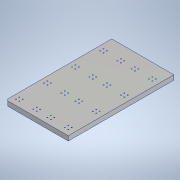
# Autodesk Inventor part: Assembly Plate
Saved by Autodesk Inventor 2022 (Build 260153000, 153)
## iProperties
Created: 2021-01-11
Part Number: Assembly Plate
Material: Aluminum 6061
Document SubType Name: Modeling
Designer: caleb
Density: 2.7 g/cm^3
Appearance: Aluminum - Flat
Author: caleb
Autodesk Inventor part; units mm, degrees
ref_plane "YZ Plane" through (0, 0, 0) normal (1, 0, 0) x (0, 1, 0)
ref_plane "XZ Plane" through (0, 0, 0) normal (0, 1, 0) x (-1, 0, 0)
ref_plane "XY Plane" through (0, 0, 0) normal (0, 0, 1) x (1, 0, 0)
sketch "Sketch1" plane through (0, 0, 0) normal (0, 1, 0) x (-1, 0, 0)
  line L0 (-63.5, 107.95) -> (63.5, 107.95)
  line L1 (63.5, 107.95) -> (63.5, -107.95)
  line L2 (63.5, -107.95) -> (-63.5, -107.95)
  line L3 (-63.5, -107.95) -> (-63.5, 107.95)
  line L4 (-63.5, 107.95) -> (63.5, -107.95) construction
  line L5 (63.5, 107.95) -> (-63.5, -107.95) construction
  point P0 (0, 0)
  dimension "d0" = 127
  dimension "d1" = 215.9
  constraints: 12 end point, 2 midpoint, 2 parallel, 1 horizontal, 1 perpendicular
  measures "d0" distance of L1.end L2.end
  measures "d1" distance of L0.end L1.end
extrude "Extrusion1" add sketch "Sketch1" along normal blind 9.525
chamfer "Chamfer1" distance 3.175 angle 45 1 edges at (-63.5, 4.7625, 107.95)
sketch "Sketch10" plane through (0, 9.525, 0) normal (0, 1, 0) x (1, 0, 0)
  circle A0 centre (-54.5, -96.95) radius 1
  circle A1 centre (-54.5, -89.95) radius 1
  circle A2 centre (-47.5, -96.95) radius 1
  circle A3 centre (-47.5, -89.95) radius 1
  line L0 (-63.5, 107.95) -> (-63.5, -104.775) projected
  line L1 (-60.325, -107.95) -> (63.5, -107.95) projected
  circle A4 centre (-54.5, -39.633) radius 1
  circle A5 centre (-54.5, -32.633) radius 1
  circle A6 centre (-47.5, -39.633) radius 1
  circle A7 centre (-47.5, -32.633) radius 1
  circle A8 centre (-54.5, 17.684) radius 1
  circle A9 centre (-54.5, 24.684) radius 1
  circle A10 centre (-47.5, 17.684) radius 1
  circle A11 centre (-47.5, 24.684) radius 1
  circle A12 centre (-54.5, 75.001) radius 1
  circle A13 centre (-54.5, 82.001) radius 1
  circle A14 centre (-47.5, 75.001) radius 1
  circle A15 centre (-47.5, 82.001) radius 1
  circle A16 centre (-18.934, -96.95) radius 1
  circle A17 centre (-18.934, -89.95) radius 1
  circle A18 centre (-11.934, -96.95) radius 1
  circle A19 centre (-11.934, -89.95) radius 1
  circle A20 centre (-18.934, -39.633) radius 1
  circle A21 centre (-18.934, -32.633) radius 1
  circle A22 centre (-11.934, -39.633) radius 1
  circle A23 centre (-11.934, -32.633) radius 1
  circle A24 centre (-18.934, 17.684) radius 1
  circle A25 centre (-18.934, 24.684) radius 1
  circle A26 centre (-11.934, 17.684) radius 1
  circle A27 centre (-11.934, 24.684) radius 1
  circle A28 centre (-18.934, 75.001) radius 1
  circle A29 centre (-18.934, 82.001) radius 1
  circle A30 centre (-11.934, 75.001) radius 1
  circle A31 centre (-11.934, 82.001) radius 1
  circle A32 centre (52.5, -96.95) radius 1
  circle A33 centre (45.5, -96.95) radius 1
  circle A34 centre (45.5, -89.95) radius 1
  circle A35 centre (52.5, -89.95) radius 1
  line L2 (63.5, -107.95) -> (63.5, 107.95) projected
  circle A36 centre (45.5, -32.633) radius 1
  circle A37 centre (45.5, -39.633) radius 1
  circle A38 centre (52.5, -39.633) radius 1
  circle A39 centre (52.5, -32.633) radius 1
  circle A40 centre (45.5, 24.684) radius 1
  circle A41 centre (45.5, 17.684) radius 1
  circle A42 centre (52.5, 17.684) radius 1
  circle A43 centre (52.5, 24.684) radius 1
  circle A44 centre (45.5, 82.001) radius 1
  circle A45 centre (45.5, 75.001) radius 1
  circle A46 centre (52.5, 75.001) radius 1
  circle A47 centre (52.5, 82.001) radius 1
  circle A48 centre (9.934, -89.95) radius 1
  circle A49 centre (9.934, -96.95) radius 1
  circle A50 centre (16.934, -96.95) radius 1
  circle A51 centre (16.934, -89.95) radius 1
  circle A52 centre (9.934, -32.633) radius 1
  circle A53 centre (9.934, -39.633) radius 1
  circle A54 centre (16.934, -39.633) radius 1
  circle A55 centre (16.934, -32.633) radius 1
  circle A56 centre (9.934, 24.684) radius 1
  circle A57 centre (9.934, 17.684) radius 1
  circle A58 centre (16.934, 17.684) radius 1
  circle A59 centre (16.934, 24.684) radius 1
  circle A60 centre (9.934, 82.001) radius 1
  circle A61 centre (9.934, 75.001) radius 1
  circle A62 centre (16.934, 75.001) radius 1
  circle A63 centre (16.934, 82.001) radius 1
  point P0 (0, 0)
  dimension "d129" = 2
  dimension "d130" = 7
  dimension "d131" = 7
  dimension "d134" = 9
  dimension "d135" = 11
  dimension "d140" = 57.317
  dimension "d143" = 35.566
  dimension "d146" = 2
  dimension "d147" = 7
  dimension "d148" = 7
  dimension "d149" = 11
  dimension "d150" = 11
  dimension "d153" = 57.317
  dimension "d156" = 35.566
  constraints: 64 centre point, 6 equal radius, 4 horizontal alignment, 4 vertical alignment, 2 horizontal, 2 vertical, 112 other
  measures "d129" diameter of A0
  measures "d130" distance of A0.centre A1.centre
  measures "d131" distance of A2.centre A0.centre
  measures "d134" distance from line of L0 A0.centre
  measures "d135" distance from line of L1 A0.centre
  measures "d140" distance of A0.centre A4.centre
  measures "d143" distance of A0.centre A16.centre
  measures "d146" diameter of A32
  measures "d147" distance of A35.centre A32.centre
  measures "d148" distance of A33.centre A32.centre
  measures "d149" distance from line of L2 A32.centre
  measures "d150" distance from line of L1 A32.centre
  measures "d153" distance of A34.centre A36.centre
  measures "d156" distance of A34.centre A48.centre
extrude "Extrusion8" cut sketch "Sketch10" against normal through all
body "Solid1"
